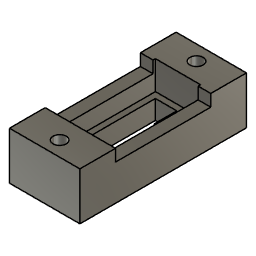
connection_PS_top v2 (Autodesk Fusion 360 design; units mm, degrees)
Autodesk Fusion 360 part; units mm, degrees
sketch "Sketch1" plane through (0, 0, 0) normal (0, 0, 1) x (1, 0, 0)
  circle A0 centre (14.6002, 31.1293) radius 1.4224
  line L0 (22.0628, -1.2359) -> (22.0962, 34.2883)
  line L1 (22.0628, -1.2359) -> (3.0128, -1.2359)
  circle A1 centre (14.5728, 1.9372) radius 1.4224
  line L2 (22.0962, 34.2883) -> (3.0462, 34.3241)
  line L3 (19.391, 6.3752) -> (6.183, 6.3752)
  line L4 (6.183, 6.3752) -> (6.183, 27.2032)
  line L5 (6.183, 27.2032) -> (19.391, 27.2032)
  line L6 (19.391, 27.2032) -> (19.391, 6.3752)
  line L7 (19.391, 6.3752) -> (6.183, 27.2032) construction
  line L8 (6.183, 6.3752) -> (19.391, 27.2032) construction
  line L9 (3.0462, 34.3241) -> (3.0128, -1.2359)
  point P0 (3.0128, 16.5441)
  point P1 (12.787, 16.7892)
  dimension "d1" = 17.78
  dimension "d3" = 2.8448
  dimension "d14" = 20.828
  dimension "d16" = 13.208
  dimension "d17" = 19.05
  dimension "d61" = 7.493
  dimension "d62" = 7.493
  constraint horizontal L1
  constraint horizontal L3
  constraint perpendicular L3 L4
  constraint parallel L3 L5
  constraint parallel L4 L6
  constraint coincident L7 P1
  constraint coincident L8 P1
  measures "d1" distance of L1.end P0
  measures "d3" diameter of A1
  measures "d14" distance of L3 L5
  measures "d16" distance of L4.end L5.end
  measures "d17" distance of L0.end L2.end
  measures "d61" distance of A1.centre L0
  measures "d62" distance of A0.centre L0
extrude "Extrude3" add sketch "Sketch1" along normal blind 10.16
sketch "Sketch5" plane through (0, 0, 0) normal (0, 0, -1) x (1, 0, 0)
  circle A0 centre (14.6002, -31.1293) radius 1.4224
  line L0 (19.391, -27.2032) -> (6.183, -27.2032)
  line L1 (6.183, -27.2032) -> (6.183, -6.3752)
  line L2 (6.183, -6.3752) -> (19.391, -6.3752)
  line L3 (19.391, -6.3752) -> (19.391, -27.2032)
  circle A1 centre (14.5728, -1.9372) radius 1.4224
  line L4 (22.0962, -34.2883) -> (22.0628, 1.2359)
  line L5 (22.0628, 1.2359) -> (3.0128, 1.2359)
  line L6 (3.0128, 1.2359) -> (3.0462, -34.3241)
  line L7 (3.0462, -34.3241) -> (22.0962, -34.2883)
  line L8 (19.391, -27.2032) -> (15.581, -27.2032)
  line L9 (15.581, -27.2032) -> (15.581, -6.3732)
  line L10 (15.581, -6.3732) -> (19.391, -6.3732)
  line L11 (19.391, -6.3732) -> (19.391, -27.2032)
  line L12 (15.3014, -12.0362) -> (15.4278, -21.1048)
  line L13 (15.4278, -21.1048) -> (19.391, -21.1048)
  line L14 (19.391, -16.7892) -> (15.3014, -12.0362) construction
  line L15 (15.4278, -21.1048) -> (19.391, -16.7892) construction
  line L16 (19.391, -12.0293) -> (15.3014, -12.0362)
  line L17 (6.183, -27.2032) -> (8.723, -27.2032)
  line L18 (8.723, -27.2032) -> (8.723, -6.3752)
  line L19 (8.723, -6.3752) -> (6.183, -6.3752)
  line L20 (6.183, -6.3752) -> (6.183, -27.2032)
  dimension "d31" = 3.81
  dimension "d36" = 2.54
  constraint horizontal L8
  constraint vertical L9
  constraint horizontal L10
  constraint vertical L11
  constraint coincident L0.start L3.end
  constraint horizontal L13
  constraint midpoint L3 L14.start
  constraint coincident L3 L13.end
  constraint coincident L3 L16.start
  constraint horizontal L17
  constraint vertical L18
  constraint horizontal L19
  constraint vertical L20
  constraint coincident L2 L18.end
  constraint coincident L0.end L1.start
  measures "d31" distance of L0.start L8.end
  measures "d36" distance of L0.end L17.end
extrude "Extrude7" add sketch "Sketch5" against normal blind 4.064 contours L0 L3 L8 L9 L11 L13 | L0 L1 L2 L17 L18 L19 L20 | L2 L3 L9 L10 L11 L16
sketch "Sketch7" plane through (3.0139, -0.0028, 0) normal (-1, 0.000941, 0) x (-0.000941, -1, 0)
  line L0 (-34.327, 0) -> (1.233, 0)
  line L1 (1.233, 0) -> (1.233, 10.16)
  line L2 (1.233, 10.16) -> (-34.327, 10.16)
  line L3 (-34.327, 10.16) -> (-34.327, 0)
  line L4 (-6.387, 7.62) -> (-26.707, 7.62)
  line L5 (-26.707, 7.62) -> (-26.707, 10.16)
  line L6 (-6.387, 10.16) -> (-6.387, 7.62)
  dimension "d65" = 20.32
  dimension "d66" = 7.62
  constraint horizontal L4
  constraint perpendicular L4 L5
  constraint parallel L5 L6
  constraint coincident L2 L5.end
  constraint coincident L2 L6.start
  measures "d65" distance of L4.start L4.end
  measures "d66" distance of L3 L5
extrude "Extrude8" cut sketch "Sketch7" against normal blind 33.02 contours L2 L4 L5 L6
extrude "Extrude9" add 1 faces at (6.183, 20.0932, 5.2493) along direction (1, 0, 0) blind 3.556
extrude "Extrude10" add 1 faces at (8.723, 20.2605, 1.3547) along direction (1, 0, 0) blind 2.286
sketch "Sketch8" plane through (0, 27.2032, 0) normal (0, -1, 0) x (1, 0, 0)
  line L0 (11.009, 4.064) -> (11.009, 0)
  line L1 (11.009, 0) -> (15.581, 0)
  line L2 (15.581, 0) -> (15.581, 4.064)
  line L3 (15.581, 4.064) -> (19.391, 4.064)
  line L4 (19.391, 4.064) -> (19.391, 10.16)
  line L5 (19.391, 10.16) -> (9.739, 10.16)
  line L6 (9.739, 10.16) -> (9.739, 4.064)
  line L7 (9.739, 4.064) -> (11.009, 4.064)
  line L8 (11.009, 4.064) -> (15.581, 4.064)
  line L9 (15.581, 4.064) -> (15.581, 0)
  line L10 (15.581, 0) -> (11.009, 0)
  line L11 (11.009, 0) -> (11.009, 4.064)
  constraint horizontal L8
  constraint vertical L9
  constraint horizontal L10
  constraint vertical L11
  constraint coincident L1.end L2.start
  constraint coincident L0.start L7.end
extrude "Extrude13" add sketch "Sketch8" along normal blind 1.27 contours L0 L1 L2 L8 L9 L10 L11
sketch "Sketch9" plane through (0, 6.3752, 0) normal (0, 1, 0) x (-1, 0, 0)
  line L0 (-11.009, 0) -> (-11.009, 4.064)
  line L1 (-11.009, 4.064) -> (-9.739, 4.064)
  line L2 (-9.739, 4.064) -> (-9.739, 10.16)
  line L3 (-9.739, 10.16) -> (-12.533, 10.16)
  line L4 (-19.391, 7.62) -> (-19.391, 4.064)
  line L5 (-19.391, 4.064) -> (-15.581, 4.064)
  line L6 (-15.581, 4.064) -> (-15.581, 0)
  line L7 (-15.581, 0) -> (-11.009, 0)
  line L8 (-15.581, 4.064) -> (-11.009, 4.064)
  line L9 (-11.009, 4.064) -> (-11.009, 0)
  line L10 (-11.009, 0) -> (-15.581, 0)
  line L11 (-15.581, 0) -> (-15.581, 4.064)
  line L12 (-12.533, 10.16) -> (-12.533, 7.62)
  line L13 (-12.533, 7.62) -> (-19.391, 7.62)
  dimension "d47" = -1.27
  constraint horizontal L8
  constraint vertical L9
  constraint horizontal L10
  constraint vertical L11
  constraint coincident L0.start L7.end
  constraint coincident L5.end L6.start
extrude "Extrude14" add sketch "Sketch9" along normal blind 1.27 contours L0 L6 L7 L8 L9 L10 L11
extrude "Extrude15" cut 1 faces at (3.0327, 19.9308, 2.54) along direction (1, -0.000941, 0) blind 3.81
extrude "Extrude16" cut 2 faces at (6.6143, 6.3807, 8.4667) (6.6143, 6.3809, 7.62) along direction (0.000941, 1, 0) blind 5.08
extrude "Extrude17" cut 2 faces at (6.8379, 14.8473, 2.54) (6.8299, 6.3809, 9.3133) along direction (1, -0.000941, 0) blind 0.2032
extrude "Extrude18" cut 1 faces at (6.9654, 6.381, 9.3133) along direction (0.000941, 1, 0) blind 3.556
